Autodesk Inventor part; units mm, degrees
(part 2 of 2)
sketch "Sketch15" plane through (-26.9555, 86.3024, -34.5) normal (-0.1460998, 0.9892699, 0) x (0.9892699, 0.1460998, 0)
  circle A0 centre (12.5463, 12.1469) radius 3
  circle A1 centre (2.955, 12.1469) radius 3
  line L0 (-0.045, 0) -> (-0.045, 15.5) projected
  ellipse E0 centre (7.2684, 6) end of major axis (2.7402, 6) minor radius 4.5 (11.1919, 8.2467) -> (11.1919, 3.7533) ccw projected
  ellipse E1 centre (17.8242, 6) end of major axis (13.296, 6) minor radius 4.5 (13.9007, 3.7533) -> (13.9007, 8.2467) ccw projected
  point P0 (14.0575, -34.5)
  dimension "d94" = 6
  dimension "d95" = 6
  dimension "d159" = 5.2779
  dimension "d160" = 5.2779
  dimension "d162" = 0
  constraints: 2 centre point, 1 tangent, 3 other
  measures "d94" diameter of A0
  measures "d95" diameter of A1
  measures "d159" horizontal distance of A0.centre point (17.824, 6)
  measures "d160" horizontal distance of A0.centre point (7.268, 6)
  measures "d162" vertical distance of A1.centre A0.centre
hole "Hole3" at (-24.0322, 86.7341, -46.6469) at (-14.5438, 88.1354, -46.6469) direction (0.1460998, -0.9892699, 0) diameter 4 depth 4 counterbore diameter 4.5 counterbore depth 0.5
sketch "Sketch17" plane through (-27, 65.2958, -50) normal (-1, 0, 0) x (0, 0, 1)
  line L0 (-0.009, 12.4464) -> (7.991, 12.4464)
  line L1 (7.991, 12.4464) -> (7.991, 18.0464)
  line L2 (7.991, 18.0464) -> (-0.009, 18.0464)
  line L3 (-0.009, 18.0464) -> (-0.009, 12.4464)
  line L4 (15.5, 12.5) -> (15.5, 12.5) projected
  line L5 (7.991, 18.0464) -> (-0.009, 12.4464)
  line L6 (-0.009, 18.0464) -> (7.991, 12.4464)
  point P0 (50, -65.2958)
  point P1 (3.991, 15.2464)
  dimension "d107" = 8
  dimension "d108" = 5.6
  constraints: 12 end point, 2 parallel, 1 horizontal, 1 midpoint, 1 perpendicular, 2 other
  measures "d107" distance of L1.end L2.end
  measures "d108" distance of L0.end L1.end
hole "Hole4" at (-27, 80.5422, -46.009) direction (1, 0, 0) diameter 4 depth 4.5 counterbore diameter 4.3 counterbore depth 0.5
ref_plane "Work Plane7" through (-13.7612, 65.7253, -40) normal (-0.0348995, 0.9993908, 0) x (-0.9993908, -0.0348995, 0)
sketch "Sketch18" plane through (-13.7612, 65.7253, -40) normal (-0.0348995, 0.9993908, 0) x (-0.9993908, -0.0348995, 0)
  circle A0 centre (0, -6.5) radius 0.75 projected
  circle A1 centre (9.6, 6.0491) radius 0.75 projected
  circle A2 centre (-9.6, 6.0491) radius 0.75 projected
  line L0 (-12.325, 5.5) -> (-12.325, -4.5) projected
  arc A3 (-12.325, -4.5) -> (-8.325, -8.5) centre (-8.325, -4.5) ccw projected
  line L1 (-8.325, -8.5) -> (8.325, -8.5) projected
  arc A4 (8.325, -8.5) -> (12.325, -4.5) centre (8.325, -4.5) ccw projected
  line L2 (12.325, -4.5) -> (12.325, 5.5) projected
  arc A5 (12.325, 5.5) -> (9.325, 8.5) centre (9.325, 5.5) ccw projected
  line L3 (9.325, 8.5) -> (-9.325, 8.5) projected
  arc A6 (-9.325, 8.5) -> (-12.325, 5.5) centre (-9.325, 5.5) ccw projected
  arc A7 (0, -0.2709) -> (0, -0.7291) centre (-5.245, -0.5) ccw projected
  arc A8 (0, -0.7291) -> (0, -0.2709) centre (5.245, -0.5) ccw projected
  line L4 (3, 8.5) -> (-3, 8.5)
  line L5 (-3, 8.5) -> (-3, 7.5)
  line L6 (-3, 7.5) -> (3, 7.5)
  line L7 (3, 7.5) -> (3, 8.5)
  line L8 (-13.7379, 10.65) -> (-10.24, 10.65) projected
  line L9 (3, 8.5) -> (3, 10.65)
  line L10 (-3, 8.5) -> (-3, 10.65)
  line L11 (-3, 10.65) -> (3, 10.65)
  point P0 (-11.4591, 40)
  dimension "d116" = 9.325
  dimension "d117" = 9.325
  dimension "d118" = 1
  dimension "d173" = 2.15
  dimension "d174" = 6
  constraints: 14 end point, 3 perpendicular, 3 point on line, 2 parallel, 1 horizontal, 1 vertical
  measures "d116" distance between parallel lines of L7 L2
  measures "d117" distance between parallel lines of L5 L0
  measures "d118" distance between parallel lines of L4 L6
  measures "d173" distance between parallel lines of L11 L4
  measures "d174" distance of L5.end L6.end
extrude "Extrusion17" cut sketch "Sketch18" along normal blind 10 contours L10 L11 L9 L3 | L3 L7 L6 L5
sketch "Sketch19" plane through (-23.8, 69.2958, -17.65) normal (0, 1, 0) x (1, 0, 0)
  circle A0 centre (4, 4.55) radius 2.25 projected
  circle A1 centre (4, 4.55) radius 3.5
  line L0 (17.8, 16.85) -> (17.8, -52.15) projected
  line L1 (6.9123, 11.7) -> (0, 5.2)
  line L2 (6.9123, 14.85) -> (0, 9.2)
  line L3 (14.5915, 0) -> (14.5915, -37.4) projected
  line L4 (12.9159, 14.85) -> (12.9159, 11.7) projected
  line L5 (12.9159, 11.7) -> (6.9123, 11.7) projected
  line L6 (6.9123, 11.7) -> (6.9123, 14.85) projected
  line L7 (1.4574, 16.85) -> (17.8, 16.85) projected
  ellipse E0 centre (0.3338, 16.3009) end of major axis (-0.9169, 16.3009) minor radius 1.25 (-0.7898, 16.85) -> (1.4574, 16.85) ccw projected
  line L8 (0, 0) -> (0, 9.2) projected
  line L9 (0, 0) -> (14.5915, 0) projected
  line L10 (14.5915, -37.4) -> (0, -37.4) projected
  line L11 (0, -37.4) -> (0, -52.15) projected
  line L12 (17.8, -52.15) -> (0, -52.15) projected
  line L13 (-3.2, 16.85) -> (-1.2, 16.85) projected
  line L14 (-3.2, 16.85) -> (-3.2, 9.2) projected
  line L15 (-3.2, 9.2) -> (0, 9.2) projected
  line L16 (6.9123, 14.85) -> (12.9159, 14.85) projected
  line L17 (-1.2, 16.85) -> (-0.7898, 16.85) projected
  point P0 (23.8, -17.65)
  point P1 (6.9123, 11.7)
  point P2 (6.9123, 14.85)
  point P3 (0, 9.2)
  point P4 (0, 5.2)
  dimension "d121" = 7
  dimension "d122" = 4
  constraints: 4 end point, 1 centre point, 1 coincident, 1 other
  measures "d121" diameter of A1
  measures "d122" distance of L2.end L1.end
extrude "Extrusion18" cut sketch "Sketch19" against normal blind 2 contours L1 A1 | A1 L1 L8 L2 L6 | L6 L16 L4 L5 picked at (1.5777, 6.7815)
mirror "Mirror2" about plane through (0, 0, 0) normal (0, 0, 1) of "Extrusion7", "Extrusion8", "Extrusion9", "Extrusion14", "Extrusion15", "Extrusion11", "Extrusion12", "Fillet1", "Extrusion13", "Hole2", "Extrusion16", "Hole3", "Hole4", "Extrusion17", "Extrusion18"
sketch "Sketch20" plane through (0, 81.4, -50) normal (1, 0, 0) x (0, 0, -1)
  line L0 (-100, 1.232) -> (-82, 1.232) projected
  arc A0 (-80, -0.768) -> (-82, 1.232) centre (-82, -0.768) ccw projected
  line L1 (-80, -0.768) -> (-80, -8.9) projected
  line L2 (-78, -10.9) -> (-22, -10.9) projected
  line L3 (-20, -8.9) -> (-20, -0.768) projected
  arc A1 (-18, 1.232) -> (-20, -0.768) centre (-18, -0.768) ccw projected
  line L4 (-18, 1.232) -> (0, 1.232) projected
  line L5 (0, 14.1) -> (0, 1.232) projected
  line L6 (0, 14.1) -> (-100, 14.1) projected
  line L7 (-100, 1.232) -> (-100, 14.1) projected
  circle A2 centre (-23.5, 3.9333) radius 3.5 projected
  circle A3 centre (-41.1667, 3.9333) radius 3.5 projected
  circle A4 centre (-58.8333, 3.9333) radius 3.5 projected
  circle A5 centre (-76.5, 3.9333) radius 3.5 projected
  circle A6 centre (-50, -3.9) radius 3.5 projected
  circle A7 centre (-50, -5.2333) radius 3.5 projected
  arc A8 (-80, -8.9) -> (-78, -10.9) centre (-78, -8.9) ccw projected
  arc A9 (-22, -10.9) -> (-20, -8.9) centre (-22, -8.9) ccw projected
  circle A10 centre (-67.6667, -3.9) radius 3.5 projected
  circle A11 centre (-67.6667, -5.2333) radius 3.5 projected
  circle A12 centre (-32.3333, -3.9) radius 3.5 projected
  circle A13 centre (-32.3333, -5.2333) radius 3.5 projected
hole "Hole5" at (0, 85.3333, 26.5) at (0, 85.3333, 8.8333) at (0, 85.3333, -26.5) at (0, 85.3333, -8.8333) at (0, 77.5, 0) direction (-1, 0, 0) diameter 2.459 depth 8.8 countersink diameter 3.5 countersink angle 90 thread size "M3x0.5" class "6H" standard "ISO Metric profile"
sketch "Sketch22" plane through (-23.8, 69.2958, -17.65) normal (0, 1, 0) x (1, 0, 0)
  circle A0 centre (14.3, -42.6439) radius 1.2295 projected
  circle A1 centre (3.7, 4.6) radius 2 projected
  circle A2 centre (7.1, -42.6439) radius 1.2295 projected
  circle A3 centre (11.3, 3.8) radius 2 projected
  circle A4 centre (11.3, 4.6) radius 2 projected
  circle A5 centre (14.3, -42.6439) radius 1.2295 projected
  point P0 (23.8, -17.65)
  point P1 (12.7, 4.55)
hole "Hole6" at (-16.7, 69.2958, 24.9939) at (-9.5, 69.2958, 24.9939) at (-20.1, 69.2958, -22.25) at (-12.5, 69.2958, -21.45) direction (0, -1, 0) diameter 3.4 depth 8.8 countersink diameter 7 countersink angle 90 clearance for "Countersunk Flat Head Screw ISO 2009/7046" size "M3" standard "ISO"
sketch "Sketch23" plane through (0, 66.2059, -50) normal (1, 0, 0) x (0, 0, -1)
  line L0 (-80, 14.4261) -> (-80, 6.2941) projected
  arc A0 (-80, 6.2941) -> (-78, 4.2941) centre (-78, 6.2941) ccw projected
  line L1 (-80.5, 15.1941) -> (-80.5, 4.2941)
  line L2 (-80.5, 4.2941) -> (-19.5, 4.2941)
  line L3 (-19.5, 4.2941) -> (-19.5, 15.1941)
  line L4 (-15.5, 3.0899) -> (-15.5, 23.1913) projected
  line L5 (-19.5, 15.1941) -> (-80.5, 15.1941)
  line L6 (-79.35, 0) -> (-79.35, -0.9101) projected
  line L7 (-20.65, -0.9101) -> (-79.35, -0.9101) projected
  line L8 (-20.65, -0.9101) -> (-20.65, 0) projected
  line L9 (-20.65, 0) -> (0, 0) projected
  line L10 (0, 15.1941) -> (0, 0) projected
  line L11 (0, 15.1941) -> (-4.1, 15.1941) projected
  line L12 (-4.1, 15.1941) -> (-4.1, 2.6261) projected
  line L13 (-4.1, 2.6261) -> (-8.6, 2.6261) projected
  line L14 (-8.6, 2.6261) -> (-8.6, 15.1941) projected
  line L15 (-8.6, 15.1941) -> (-91.4, 15.1941) projected
  line L16 (-91.4, 15.1941) -> (-91.4, 2.6261) projected
  line L17 (-91.4, 2.6261) -> (-95.9, 2.6261) projected
  line L18 (-95.9, 2.6261) -> (-95.9, 15.1941) projected
  line L19 (-95.9, 15.1941) -> (-100, 15.1941) projected
  line L20 (-100, 15.1941) -> (-100, 0) projected
  line L21 (-100, 0) -> (-79.35, 0) projected
  line L22 (-78, 4.2941) -> (-22, 4.2941) projected
  circle A1 centre (-67.6667, 9.9608) radius 3.5 projected
  circle A2 centre (-76.5, 19.1274) radius 3.5 projected
  circle A3 centre (-58.8333, 19.1274) radius 3.5 projected
  circle A4 centre (-41.1667, 19.1274) radius 3.5 projected
  circle A5 centre (-23.5, 19.1274) radius 3.5 projected
  line L23 (-18, 16.4261) -> (0, 16.4261) projected
  line L24 (0, 29.2941) -> (0, 16.4261) projected
  line L25 (-100, 16.4261) -> (-100, 29.2941) projected
  line L26 (-100, 16.4261) -> (-82, 16.4261) projected
  arc A6 (-22, 4.2941) -> (-20, 6.2941) centre (-22, 6.2941) ccw projected
  line L27 (-20, 6.2941) -> (-20, 14.4261) projected
  arc A7 (-18, 16.4261) -> (-20, 14.4261) centre (-18, 14.4261) ccw projected
  line L28 (0, 29.2941) -> (-100, 29.2941) projected
  arc A8 (-80, 14.4261) -> (-82, 16.4261) centre (-82, 14.4261) ccw projected
  circle A9 centre (-50, 9.9608) radius 3.5 projected
  circle A10 centre (-32.3333, 9.9608) radius 3.5 projected
  point P0 (-50, -66.2059)
  point P1 (-20, 15.1941)
  point P2 (-80, 9.2941)
  point P3 (-98, 16.4261)
  point P4 (-100, 18.4261)
  point P5 (-20, 12.9261)
  point P6 (-2, 16.4261)
  point P7 (0, 18.4261)
  dimension "d187" = 0
  dimension "d188" = 0.5
  dimension "d189" = 0.5
  dimension "d190" = 0
  dimension "d191" = 19.5
  dimension "d192" = 19.5
  constraints: 8 end point, 2 horizontal, 1 parallel, 1 vertical, 3 other
  measures "d187" vertical extent of L5
  measures "d188" distance from line of point (-80, 9.294) L1
  measures "d189" distance from line of point (-20, 15.194) L3
  measures "d190" distance between parallel lines of L2 L22
  measures "d191" distance between parallel lines of L20 L1
  measures "d192" distance between parallel lines of L10 L3
ref_plane "Work Plane11" through (-3, 77, -50) normal (-1, 0, 0) x (0, 0, 1)
extrude "Extrusion19" cut sketch "Sketch23" against normal up to surface (3 mm away) contours A8 L5 A7 L27 A6 L2 A0 L0 | L0 A0 L2 L1 L5 A8 | L5 L3 L2 A6 L27 A7 | A1 | A9 | A10
body "Solid2"
